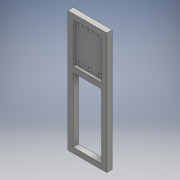
# Autodesk Inventor part: framesideRight
Saved by Autodesk Inventor 2016 (Build 200138000, 138)
## iProperties
Created: 2016-05-18
Part Number: framesideRight
Material: Generic
Document SubType Name: Modeling
Designer: hesaon
Density: 1 g/cm^3
Appearance: Default
Author: hesaon
Autodesk Inventor part; units mm, degrees
ref_plane "YZ Plane" through (0, 0, 0) normal (1, 0, 0) x (0, 1, 0)
ref_plane "XZ Plane" through (0, 0, 0) normal (0, 1, 0) x (-1, 0, 0)
ref_plane "XY Plane" through (0, 0, 0) normal (0, 0, 1) x (1, 0, 0)
sketch "Sketch1" plane through (0, 0, 0) normal (0, 1, 0) x (-1, 0, 0)
  line L0 (0, 0) -> (58, 0)
  line L1 (58, 0) -> (58, -180)
  line L2 (58, -180) -> (0, -180)
  line L3 (0, -180) -> (0, 0)
  line L4 (50, -8) -> (8, -8)
  line L5 (8, -172) -> (50, -172)
  line L6 (50, -68) -> (8, -68)
  line L7 (50, -76) -> (8, -76)
  line L8 (50, -172) -> (50, -76)
  line L9 (50, -68) -> (50, -8)
  line L10 (8, -8) -> (8, -68)
  line L11 (8, -76) -> (8, -172)
  dimension "d0" = 58
  dimension "d1" = 180
  dimension "d2" = 164
  dimension "d3" = 42
  dimension "d4" = 8
  dimension "d5" = 8
  dimension "d6" = 60
  dimension "d7" = 8
  dimension "d8" = 8
  dimension "d9" = 8
  constraints: 24 end point, 7 parallel, 7 perpendicular, 2 horizontal
  measures "d0" distance of L1.end L2.end
  measures "d1" distance of L0.end L1.end
  measures "d2" distance of L5.end L4.start
  measures "d3" distance of L5.start L5.end
  measures "d4" distance from line of L2 L5.start
  measures "d5" distance from line of L1 L5.end
  measures "d6" distance of L4.end L6.end
  measures "d7" distance of L7.end L6.end
  measures "d8" distance between parallel lines of L0 L4
  measures "d9" distance from line of L3 L4.end
extrude "Extrusion1" add sketch "Sketch1" along normal blind 8
sketch "Sketch2" plane through (0, 8, 0) normal (0, 1, 0) x (1, 0, 0)
  circle A0 centre (-44, 13) radius 2.1
  circle A1 centre (-29, 13) radius 2.1
  circle A2 centre (-14, 13) radius 2.1
  circle A3 centre (-44, 63) radius 2.1
  circle A4 centre (-29, 63) radius 2.1
  circle A5 centre (-14, 63) radius 2.1
  line L0 (-8, 8) -> (-8, 68) projected
  line L1 (-8, 8) -> (-50, 8) projected
  line L2 (-8, 68) -> (-50, 68) projected
  line L3 (-50, 8) -> (-8, 8) projected
  line L4 (-50, 8) -> (-50, 68)
  line L5 (-50, 8) -> (-50, 68) projected
  line L6 (-50, 8) -> (-8, 8)
  line L7 (-8, 68) -> (-8, 8) projected
  line L8 (-8, 8) -> (-8, 68)
  line L9 (-8, 68) -> (-50, 68)
  dimension "d12" = 4.2
  dimension "d13" = 4.2
  dimension "d15" = 4.2
  dimension "d16" = 4.2
  dimension "d17" = 4.2
  dimension "d42" = 21
  dimension "d43" = 21
  dimension "d44" = 15
  dimension "d45" = 15
  dimension "d46" = 15
  dimension "d47" = 15
  dimension "d48" = 4.2
  dimension "d49" = 5
  dimension "d50" = 5
  dimension "d51" = 5
  dimension "d52" = 5
  dimension "d53" = 5
  constraints: 8 end point, 6 centre point, 2 perpendicular, 1 collinear, 1 vertical
  measures "d12" diameter of A0
  measures "d13" diameter of A1
  measures "d15" diameter of A3
  measures "d16" diameter of A4
  measures "d17" diameter of A5
  measures "d42" distance from line of L0 A1.centre
  measures "d43" distance from line of L0 A4.centre
  measures "d44" distance of A4.centre A5.centre
  measures "d45" distance of A4.centre A3.centre
  measures "d46" distance of A1.centre A0.centre
  measures "d47" distance of A2.centre A1.centre
  measures "d48" diameter of A2
  measures "d49" distance from line of L1 A1.centre
  measures "d50" distance from line of L2 A4.centre
  measures "d51" distance from line of L2 A5.centre
  measures "d52" distance from line of L2 A3.centre
  measures "d53" distance from line of L1 A0.centre
extrude "Extrusion2" add sketch "Sketch2" against normal blind 4
body "Solid1"
